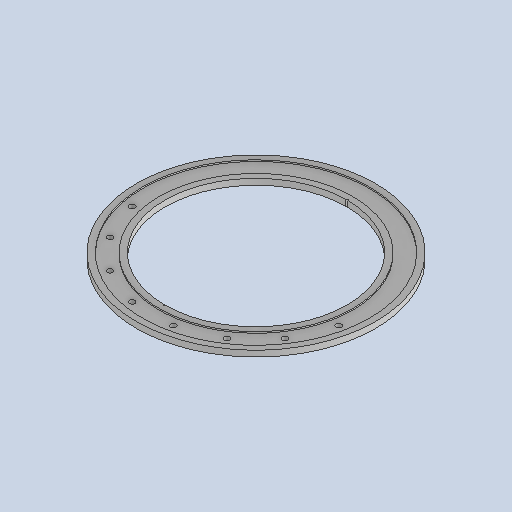
# Autodesk Inventor part: ДМФ 022 кольцо прижимное корма v2.0
Saved by Autodesk Inventor 2025 (Build 290162010, 162A)
## iProperties
Created: 2024-04-23
Part Number: ДМФ 022 кольцо прижимное корма v2.0
Material: Generic
Document SubType Name: Sheet Metal
Designer: admin
Density: 1 g/cm^3
Appearance: Default
Flat Pattern Width: 60.2 cm
Flat Pattern Length: 60.2 cm
Flat Pattern Area: 3624.04 cm^2
Sheet Metal Rule: Default
Sheet Metal Width: 602,000 mm
Sheet Metal Length: 602,000 mm
Sheet Metal Area: 362404,000 mm^2
Stock Number: ДМФ 022 кольцо прижимное корма внутреннее
Author: admin
Autodesk Inventor part; units mm, degrees
note: some values were not read from the file. Chosen so that the rebuilt part matches the saved one: pattern direction of "Circular Pattern2".
ref_plane "YZ Plane" through (0, 0, 0) normal (1, 0, 0) x (0, 1, 0)
ref_plane "XZ Plane" through (0, 0, 0) normal (0, 1, 0) x (-1, 0, 0)
ref_plane "XY Plane" through (0, 0, 0) normal (0, 0, 1) x (1, 0, 0)
sketch "Sketch1" plane through (0, 0, 0) normal (0, 0, 1) x (1, 0, 0)
  circle A0 centre (0, 0) radius 229
  circle A1 centre (0, 0) radius 301
  circle A2 centre (0, 0) radius 265 construction
  line L0 (0, 229) -> (0, 301) construction
  point P0 (0, 265)
  dimension "d17" = 530
  dimension "d18" = 72
  constraints: 4 vertical alignment, 3 coincident, 2 end point, 1 midpoint, 1 vertical, 6 other
  measures "d18" distance of L0.start L0.end
extrude "Extrusion1" add sketch "Sketch1" along normal blind 15
sketch "Sketch2" plane through (0, 0, 15) normal (0, 0, 1) x (1, 0, 0)
  circle A0 centre (0, 0) radius 301 construction
  circle A1 centre (0, 0) radius 229 construction
  line L0 (0, 286) -> (0, 244) construction
  line L1 (0, 229) -> (0, 0) construction
  circle A2 centre (0, 0) radius 244
  circle A3 centre (0, 0) radius 286
  circle A4 centre (0, 0) radius 265 construction
  point P0 (0, 265)
  dimension "d19" = 530
  dimension "d4" = 42
  constraints: 5 vertical alignment, 4 end point, 3 coincident, 2 vertical, 1 midpoint, 7 other
  measures "d4" distance of L0.start L0.end
extrude "Extrusion2" cut sketch "Sketch2" against normal blind 3.5
sketch "Sketch3" plane through (0, 0, 0) normal (0, 0, 1) x (1, 0, 0)
  circle A0 centre (0, 0) radius 229 construction
  circle A1 centre (0, 0) radius 301 construction
  circle A2 centre (0, 0) radius 244 projected
  circle A3 centre (0, 0) radius 286 projected
  circle A4 centre (0, 0) radius 301 projected
  line L0 (0, 0) -> (0, -301) construction
  line L1 (0, 0) -> (58.7222, -295.2164) construction
  line L2 (47.602, -239.3116) -> (55.7958, -280.5046) construction
  circle A5 centre (51.6989, -259.9081) radius 7
  dimension "d20" = 11.25
  dimension "d21" = 14
  constraints: 6 end point, 2 point on circle, 2 point on line, 1 centre point, 1 midpoint, 1 vertical, 4 other
  measures "d20" angle of L1 L0
  measures "d21" diameter of A5
extrude "Extrusion3" cut sketch "Sketch3" along normal through all contours A5
pattern_circular "Circular Pattern2" count 8 over 157.5 about axis through (0, 0, 0) along (0, 0, -1) of "Extrusion3" both ways yes
sketch "Sketch5" plane through (0, 0, 0) normal (0, 0, -1) x (-1, 0, 0)
  circle A0 centre (0, 0) radius 301 projected
  circle A1 centre (0, 0) radius 229 projected
  line L0 (0, 0) -> (0, 229) construction
  arc A2 (2.5, 228.9864) -> (-2.5, 228.9864) centre (0, 229) ccw
  dimension "d40" = 5
  constraints: 5 point on circle, 2 end point, 1 centre point, 1 coincident, 1 vertical
  measures "d40" diameter of A2
extrude "Extrusion4" cut sketch "Sketch5" against normal through all contours A1 A2
mirror "Mirror1" about plane through (0, 0, 0) normal (0, 1, 0) of "Extrusion4"
equation "\"d17\" = Шпил_пласт_КОРМА_диам_центров"
equation "\"d19\" = Шпил_пласт_КОРМА_диам_центров"
equation "\"BendReliefDepth\" = 0.5 * Thickness"
equation "\"Шпил_пласт_КОРМА_диам_центров\" = 530"
equation "\"Thickness\" = 10"
body "Solid1"
